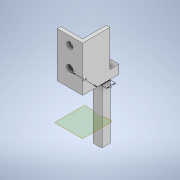
# Autodesk Inventor part: Part2
Saved by Autodesk Inventor 2020 (Build 240168000, 168)
## iProperties
Created: 2023-01-29
Part Number: Part2
Material: Generic
Document SubType Name: Modeling
Designer: ma203
Density: 1 g/cm^3
Appearance: Default
Author: ma203
## iProperties of the stored document _3DPrint.ipt
Part Number: _3DPrint
Material: Generic
Document SubType Name: Modeling
Designer: ma203
Appearance: Default
Author: ma203
Autodesk Inventor part; units mm, degrees
ref_plane "YZ Plane" through (0, 0, 0) normal (1, 0, 0) x (0, 1, 0)
ref_plane "XZ Plane" through (0, 0, 0) normal (0, 1, 0) x (-1, 0, 0)
ref_plane "XY Plane" through (0, 0, 0) normal (0, 0, 1) x (1, 0, 0)
sketch "Sketch1" plane through (0, 0, 0) normal (0, 1, 0) x (-1, 0, 0)
  line L0 (0, 0) -> (0, -13)
  line L1 (0, -13) -> (-2, -13)
  line L2 (-2, -13) -> (-2, 2)
  line L3 (-2, 2) -> (12, 2)
  line L4 (12, 2) -> (12, -13)
  line L5 (12, -13) -> (10, -13)
  line L6 (10, -13) -> (10, 0)
  line L7 (10, 0) -> (0, 0)
  dimension "d0" = 13
  dimension "d1" = 2
  dimension "d2" = 15
  dimension "d3" = 14
  dimension "d4" = 2
  dimension "d5" = 13
  constraints: 16 end point, 4 perpendicular, 2 point on line, 1 parallel, 1 vertical
  measures "d0" distance of L0.start L0.end
  measures "d1" distance of L0.end L1.end
  measures "d2" distance of L1.end L2.end
  measures "d3" distance of L2.end L3.end
  measures "d4" distance of L4.end L5.end
  measures "d5" distance of L5.end L6.end
extrude "Extrusion1" add sketch "Sketch1" along normal blind 20
sketch "Sketch2" plane through (-12, 0, 2) normal (0, 0, 1) x (1, 0, 0)
  line L0 (0, 20) -> (14, 20) projected
  line L1 (7, 20) -> (7, 0)
  line L2 (12, 0) -> (2, 0) projected
  line L3 (7, 0) -> (7, 4.5)
  circle A0 centre (7, 4.5) radius 1.75
  line L4 (7, 4.5) -> (7, 15.5)
  circle A1 centre (7, 15.5) radius 1.75
  dimension "d8" = 4.5
  dimension "d9" = 3.5
  dimension "d10" = 11
  dimension "d11" = 3.5
  constraints: 6 end point, 2 centre point, 2 coincident, 2 midpoint, 2 point on line
  measures "d8" distance of L1.end L3.end
  measures "d9" diameter of A0
  measures "d10" distance of L4.start L4.end
  measures "d11" diameter of A1
extrude "Extrusion2" cut sketch "Sketch2" against normal blind 20
sketch "Sketch3" plane through (0, 0, 0) normal (0, -1, 0) x (1, 0, 0)
  line L0 (-12, 2) -> (2, 2) projected
  line L1 (-12, -13) -> (-12, 2) projected
  line L2 (2, 2) -> (-12, 2)
  line L3 (-12, 2) -> (-12, -13)
  line L4 (-12, -13) -> (2, -13)
  line L5 (2, -13) -> (2, 2)
  point P0 (0, 0)
  constraints: 8 end point, 2 parallel, 1 horizontal, 1 perpendicular
extrude "Extrusion3" add sketch "Sketch3" along normal blind 5
sketch "Sketch4" plane through (0, -5, 0) normal (0, -1, 0) x (1, 0, 0)
  line L0 (-12, -13) -> (2, -13) projected
  line L1 (2, -13) -> (-12, -13)
  line L2 (-12, -13) -> (-12, -8)
  line L3 (-12, -8) -> (2, -8)
  line L4 (2, -8) -> (2, -13)
  point P0 (0, 0)
  dimension "d16" = 14
  dimension "d17" = 5
  constraints: 8 end point, 2 parallel, 1 horizontal, 1 perpendicular
  measures "d16" distance of L2.end L3.end
  measures "d17" distance of L3.end L0.end
ref_plane "Work Plane1" through (0, -25, 0) normal (0, -1, 0) x (1, 0, 0)
sketch "Sketch5" plane through (0, -25, 0) normal (0, -1, 0) x (1, 0, 0)
  line L0 (2, -8) -> (2, -13) projected
  line L1 (-12, -13) -> (2, -13) projected
  line L2 (-5, -13) -> (-5, 2)
  line L3 (2, 2) -> (-12, 2) projected
  line L4 (-5, -13) -> (-2.5, -13)
  line L5 (-10, -13) -> (0, -13) projected
  line L6 (-2.5, -13) -> (-2.5, -18)
  line L7 (-2.5, -18) -> (-7.5, -18)
  line L8 (-7.5, -18) -> (-7.5, -13)
  line L9 (-2.5, -13) -> (-7.5, -13)
  line L10 (-5, -13) -> (-5, -25.5)
  arc A0 (-2.4988, -13.2528) -> (-5, -13) centre (-5, -25.5) ccw
  arc A1 (-5, -13) -> (-7.5, -13.2526) centre (-5, -25.5) ccw
  point P0 (0, 0)
  point P1 (-2.5, -13.2526)
  dimension "d25" = 2.5
  dimension "d26" = 5
  dimension "d27" = 5
  dimension "d31" = 12.5
  constraints: 14 end point, 5 point on circle, 4 perpendicular, 3 point on line, 2 centre point, 2 coincident, 2 midpoint, 1 vertical
  measures "d25" distance of L2.start L4.end
  measures "d26" distance of L4.end L6.end
  measures "d27" distance of L6.end L7.end
  measures "d31" distance of L2.start L10.end
extrude "Extrusion4" add sketch "Sketch5" against normal blind 20 contours A0 L6 L7 L10 | L10 L7 L8 A1
sketch "Sketch6" plane through (2, 20, -13) normal (0, 0, -1) x (-1, 0, 0)
  line L0 (0, -25) -> (0, 0) projected
  line L1 (14, -25) -> (7, -25) projected
  line L2 (0, -20) -> (14, -20)
  line L3 (14, -20) -> (14, -25)
  line L4 (14, -25) -> (0, -25)
  line L5 (0, -25) -> (0, -20)
  point P0 (2, -20)
  point P1 (9.5, -25)
  point P2 (9.5, -25)
  constraints: 8 end point, 2 parallel, 1 horizontal, 1 perpendicular, 1 point on line
extrude "Extrusion5" add sketch "Sketch6" along normal up to surface (5 mm away)
fillet "Fillet1" radius 2 1 edges at (-5, -5, -13)
sketch "Sketch9" plane through (0, -25, 0) normal (0, -1, 0) x (1, 0, 0)
  arc A0 (-2.5, -13.2526) -> (-7.5, -13.2526) centre (-5, -25.5) ccw projected
  line L0 (-7.5, -13.2526) -> (-7.5, -18) projected
  line L1 (-7.5, -18) -> (-2.5, -18) projected
  line L2 (-2.5, -18) -> (-2.5, -13.2526) projected
  line L3 (-2.5, -18) -> (-2.5, -13.2526)
  line L4 (-2.5, -11.2171) -> (-2.5, -18) projected
  line L5 (-2.5, -18) -> (-7.5, -18)
  line L6 (2, -18) -> (-12, -18) projected
  line L7 (-7.5, -18) -> (-7.5, -13.2526)
  point P0 (0, 0)
  constraints: 6 end point, 3 collinear
extrude "Extrusion7" add sketch "Sketch9" along normal blind 15
sketch "Sketch10" plane through (-10, 20, -13) normal (0, 0, -1) x (-1, 0, 0)
  line L0 (2, -20) -> (2, 0) projected
  line L1 (0, -20) -> (0, 0) projected
  line L2 (2, 0) -> (0, 0)
  line L3 (0, 0) -> (0, -20)
  line L4 (0, -20) -> (2, -20)
  line L5 (2, -20) -> (2, 0)
  point P0 (-10, -20)
  constraints: 8 end point, 2 parallel, 1 horizontal, 1 perpendicular
extrude "Extrusion8" cut sketch "Sketch10" against normal up to surface (13 mm away)
body "Solid1"
